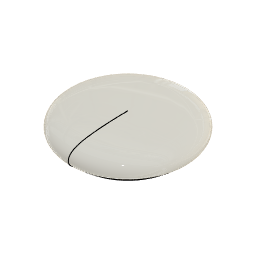
airtag (Autodesk Fusion 360 design; units mm, degrees)
Autodesk Fusion 360 part; units mm, degrees
sketch "airtag_guidelines" plane through (0, 0, 0) normal (1, 0, 0) x (0, 1, 0)
  spline S0 degree 5 poles (15.93, 7.98) (15.8968, 7.9797) (15.8305, 7.9792) (15.731, 7.9782) (15.5984, 7.9768) (15.4326, 7.9748) (15.2668, 7.9725) (15.1011, 7.97) (14.9353, 7.9675) (14.7696, 7.9651) (14.6038, 7.963) (14.438, 7.9613) (14.2722, 7.9599) (14.1063, 7.9589) (13.9405, 7.9579) (13.7747, 7.9563) (13.6089, 7.954) (13.4432, 7.9504) (13.2776, 7.9456) (13.112, 7.9397) (12.9463, 7.9332) (12.7805, 7.9265) (12.6146, 7.9201) (12.4485, 7.9141) (12.2825, 7.9085) (12.1166, 7.903) (11.951, 7.897) (11.7857, 7.8905) (11.6209, 7.883) (11.4563, 7.8749) (11.292, 7.8664) (11.1275, 7.858) (10.9629, 7.85) (10.7979, 7.8425) (10.6324, 7.8353) (10.4666, 7.8278) (10.3005, 7.8198) (10.1343, 7.8106) (9.9681, 7.8001) (9.802, 7.7884) (9.6363, 7.7759) (9.471, 7.7631) (9.3062, 7.7504) (9.1418, 7.7381) (8.9776, 7.7262) (8.8134, 7.7145) (8.6489, 7.7027) (8.484, 7.6905) (8.3185, 7.6776) (8.1528, 7.664) (7.9869, 7.6499) (7.8213, 7.6354) (7.6561, 7.6206) (7.4914, 7.6056) (7.3272, 7.5903) (7.1632, 7.5745) (6.9991, 7.5581) (6.8346, 7.5407) (6.6697, 7.5224) (6.5043, 7.5031) (6.3387, 7.483) (6.1733, 7.4623) (6.0081, 7.4411) (5.8435, 7.4197) (5.6793, 7.3981) (5.5155, 7.3762) (5.3518, 7.354) (5.1881, 7.3313) (5.0242, 7.3079) (4.8602, 7.2835) (4.6963, 7.2579) (4.5325, 7.2308) (4.369, 7.2021) (4.2061, 7.1716) (4.0436, 7.1393) (3.8817, 7.1053) (3.7201, 7.0696) (3.5589, 7.0325) (3.3981, 6.9939) (3.2375, 6.9538) (3.0773, 6.9121) (2.9176, 6.8686) (2.7585, 6.8231) (2.6001, 6.7754) (2.4426, 6.7249) (2.2861, 6.6715) (2.1309, 6.6147) (1.977, 6.5541) (1.8247, 6.4894) (1.6742, 6.4204) (1.5257, 6.3469) (1.3795, 6.2687) (1.2359, 6.1854) (1.0956, 6.0968) (0.9593, 6.0023) (0.8277, 5.9012) (0.7019, 5.793) (0.583, 5.6772) (0.472, 5.5536) (0.37, 5.4222) (0.2781, 5.2835) (0.1973, 5.138) (0.1288, 4.9864) (0.0733, 4.8296) (0.0316, 4.6687) (0.0046, 4.5046) (-0.0074, 4.3386) (-0.004, 4.172) (0.0148, 4.0061) (0.0489, 3.8424) (0.0977, 3.6825) (0.1605, 3.5277) (0.2364, 3.3793) (0.3243, 3.238) (0.4228, 3.1043) (0.5307, 2.9782) (0.6465, 2.8595) (0.7691, 2.7478) (0.8975, 2.643) (1.0309, 2.5447) (1.1691, 2.4529) (1.2832, 2.3846) (1.3708, 2.3362) (1.4301, 2.3052) (1.46, 2.29) knots 0 0 0 0 0 0 0.00833333 0.01666667 0.025 0.03333333 0.04166667 0.05 0.05833333 0.06666667 0.075 0.08333333 0.09166667 0.1 0.10833333 0.11666667 0.125 0.13333333 0.14166667 0.15 0.15833333 0.16666667 0.175 0.18333333 0.19166667 0.2 0.20833333 0.21666667 0.225 0.23333333 0.24166667 0.25 0.25833333 0.26666667 0.275 0.28333333 0.29166667 0.3 0.30833333 0.31666667 0.325 0.33333333 0.34166667 0.35 0.35833333 0.36666667 0.375 0.38333333 0.39166667 0.4 0.40833333 0.41666667 0.425 0.43333333 0.44166667 0.45 0.45833333 0.46666667 0.475 0.48333333 0.49166667 0.5 0.50833333 0.51666667 0.525 0.53333333 0.54166667 0.55 0.55833333 0.56666667 0.575 0.58333333 0.59166667 0.6 0.60833333 0.61666667 0.625 0.63333333 0.64166667 0.65 0.65833333 0.66666667 0.675 0.68333333 0.69166667 0.7 0.70833333 0.71666667 0.725 0.73333333 0.74166667 0.75 0.75833333 0.76666667 0.775 0.78333333 0.79166667 0.8 0.80833333 0.81666667 0.825 0.83333333 0.84166667 0.85 0.85833333 0.86666667 0.875 0.88333333 0.89166667 0.9 0.90833333 0.91666667 0.925 0.93333333 0.94166667 0.95 0.95833333 0.96666667 0.975 0.98333333 0.99166667 1 1 1 1 1 1
  spline S1 degree 5 poles (3.21, 0.88) (3.2486, 0.8746) (3.3257, 0.8637) (3.4417, 0.8476) (3.5967, 0.8264) (3.791, 0.8004) (3.9858, 0.7748) (4.1811, 0.7497) (4.3768, 0.7251) (4.5727, 0.7008) (4.7684, 0.6769) (4.9639, 0.6533) (5.1589, 0.6301) (5.3535, 0.6071) (5.5478, 0.5846) (5.742, 0.5624) (5.9363, 0.5408) (6.131, 0.5198) (6.3261, 0.4992) (6.5217, 0.4791) (6.7176, 0.4592) (6.9136, 0.4395) (7.1096, 0.42) (7.3055, 0.4006) (7.5011, 0.3817) (7.6968, 0.3634) (7.8925, 0.346) (8.0885, 0.3298) (8.2846, 0.3148) (8.4808, 0.3007) (8.6769, 0.2872) (8.8728, 0.2738) (9.0682, 0.2602) (9.2632, 0.2462) (9.4579, 0.2319) (9.6524, 0.2175) (9.847, 0.2033) (10.0419, 0.1897) (10.2372, 0.1768) (10.4329, 0.1645) (10.6291, 0.1527) (10.8255, 0.1412) (11.0219, 0.1299) (11.2183, 0.1186) (11.4145, 0.1076) (11.6105, 0.0972) (11.8063, 0.0878) (12.002, 0.0796) (12.1977, 0.0726) (12.3934, 0.0666) (12.5894, 0.0612) (12.7857, 0.0558) (12.9824, 0.05) (13.1795, 0.0438) (13.3769, 0.0372) (13.5743, 0.0307) (13.7717, 0.0247) (13.9688, 0.0197) (14.1655, 0.0159) (14.3618, 0.0134) (14.5578, 0.0118) (14.7536, 0.0108) (14.9493, 0.01) (15.1451, 0.0091) (15.341, 0.0078) (15.5371, 0.0059) (15.6942, 0.0038) (15.812, 0.002) (15.8907, 0.0007) (15.93, 0) knots 0 0 0 0 0 0 0.01538462 0.03076923 0.04615385 0.06153846 0.07692308 0.09230769 0.10769231 0.12307692 0.13846154 0.15384615 0.16923077 0.18461538 0.2 0.21538462 0.23076923 0.24615385 0.26153846 0.27692308 0.29230769 0.30769231 0.32307692 0.33846154 0.35384615 0.36923077 0.38461538 0.4 0.41538462 0.43076923 0.44615385 0.46153846 0.47692308 0.49230769 0.50769231 0.52307692 0.53846154 0.55384615 0.56923077 0.58461538 0.6 0.61538462 0.63076923 0.64615385 0.66153846 0.67692308 0.69230769 0.70769231 0.72307692 0.73846154 0.75384615 0.76923077 0.78461538 0.8 0.81538462 0.83076923 0.84615385 0.86153846 0.87692308 0.89230769 0.90769231 0.92307692 0.93846154 0.95384615 0.96923077 0.98461538 1 1 1 1 1 1
  line L0 (3.205, 1.89) -> (15.93, 1.89)
  line L1 (15.93, 1.89) -> (15.93, 0.88)
  line L2 (15.93, 0.88) -> (3.205, 0.88)
  line L3 (3.155, 0.93) -> (3.155, 1.84)
  line L4 (15.93, 7.98) -> (15.93, 0)
  line L5 (4.375, 2.29) -> (15.93, 2.29)
  line L6 (15.93, 2.29) -> (15.93, 1.89)
  line L7 (15.93, 1.89) -> (4.375, 1.89)
  line L8 (4.375, 1.89) -> (4.375, 2.29)
  line L9 (1.46, 2.29) -> (4.375, 2.29)
  line L10 (3.205, 1.89) -> (3.155, 1.84)
  line L11 (3.205, 0.88) -> (3.155, 0.93)
  point P0 (15.93, 0)
  point P1 (14.95, 0.01)
  point P2 (13.97, 0.02)
  point P3 (12.98, 0.05)
  point P4 (12, 0.08)
  point P5 (11.02, 0.13)
  point P6 (10.04, 0.19)
  point P7 (9.07, 0.26)
  point P8 (0.77, 2.75)
  point P9 (1.46, 2.29)
  point P10 (3.21, 0.88)
  point P11 (4.18, 0.75)
  point P12 (5.16, 0.63)
  point P13 (6.13, 0.52)
  point P14 (7.11, 0.42)
  point P15 (8.09, 0.33)
  point P16 (13.44, 7.95)
  point P17 (14.27, 7.96)
  point P18 (0.58, 5.67)
  point P19 (0.13, 4.98)
  point P20 (0.24, 3.38)
  point P21 (0, 4.17)
  point P22 (15.93, 7.98)
  point P23 (15.1, 7.97)
  point P24 (6.83, 7.54)
  point P25 (7.65, 7.62)
  point P26 (8.48, 7.69)
  point P27 (9.3, 7.75)
  point P28 (10.13, 7.81)
  point P29 (10.96, 7.85)
  point P30 (11.78, 7.89)
  point P31 (12.61, 7.92)
  point P32 (1.97, 6.55)
  point P33 (2.75, 6.82)
  point P34 (3.55, 7.03)
  point P35 (4.36, 7.2)
  point P36 (5.18, 7.33)
  point P37 (6, 7.44)
  point P38 (1.23, 6.18)
  point P39 (15.1, 7.97)
  point P40 (14.27, 7.96)
  point P41 (13.44, 7.95)
  point P42 (12.61, 7.92)
  point P43 (11.78, 7.89)
  point P44 (10.96, 7.85)
  point P45 (10.13, 7.81)
  point P46 (9.3, 7.75)
  point P47 (8.48, 7.69)
  point P48 (7.65, 7.62)
  point P49 (6.83, 7.54)
  point P50 (6, 7.44)
  point P51 (5.18, 7.33)
  point P52 (4.36, 7.2)
  point P53 (3.55, 7.03)
  point P54 (2.75, 6.82)
  point P55 (1.97, 6.55)
  point P56 (1.23, 6.18)
  point P57 (0.58, 5.67)
  point P58 (0.13, 4.98)
  point P59 (0, 4.17)
  point P60 (0.24, 3.38)
  point P61 (0.77, 2.75)
  point P62 (4.18, 0.75)
  point P63 (5.16, 0.63)
  point P64 (6.13, 0.52)
  point P65 (7.11, 0.42)
  point P66 (8.09, 0.33)
  point P67 (9.07, 0.26)
  point P68 (10.04, 0.19)
  point P69 (11.02, 0.13)
  point P70 (12, 0.08)
  point P71 (12.98, 0.05)
  point P72 (13.97, 0.02)
  point P73 (14.95, 0.01)
  point P74 (3.155, 1.89)
  point P75 (3.155, 0.88)
  dimension "d4_1" = 15.93
  dimension "d5_1" = 14.95
  dimension "d6_1" = 0.01
  dimension "d7_1" = 13.97
  dimension "d8_1" = 0.02
  dimension "d9_1" = 12.98
  dimension "d10_1" = 0.05
  dimension "d11_1" = 12
  dimension "d12_1" = 0.08
  dimension "d13_1" = 11.02
  dimension "d14_1" = 0.13
  dimension "d15_1" = 10.04
  dimension "d16_1" = 0.19
  dimension "d17_1" = 9.07
  dimension "d18_1" = 0.26
  dimension "d19_1" = 8.09
  dimension "d20_1" = 0.33
  dimension "d21_1" = 7.11
  dimension "d22_1" = 0.42
  dimension "d23_1" = 6.13
  dimension "d24_1" = 0.52
  dimension "d25_1" = 5.16
  dimension "d26_1" = 0.63
  dimension "d27_1" = 4.18
  dimension "d28_1" = 0.75
  dimension "d29_1" = 3.21
  dimension "d30_1" = 0.88
  dimension "d31_1" = 1.46
  dimension "d32_1" = 2.29
  dimension "d33_1" = 0.77
  dimension "d34_1" = 2.75
  dimension "d35_1" = 0.24
  dimension "d36_1" = 3.38
  dimension "d37_1" = 4.17
  dimension "d38_1" = 0.13
  dimension "d39_1" = 4.98
  dimension "d40_1" = 0.58
  dimension "d41_1" = 5.67
  dimension "d42_1" = 15.93
  dimension "d43_1" = 7.98
  dimension "d44_1" = 15.1
  dimension "d45_1" = 7.97
  dimension "d46_1" = 14.27
  dimension "d47_1" = 7.96
  dimension "d48_1" = 13.44
  dimension "d49_1" = 7.95
  dimension "d50_1" = 12.61
  dimension "d51_1" = 7.92
  dimension "d52_1" = 11.78
  dimension "d53_1" = 7.89
  dimension "d54_1" = 10.96
  dimension "d55_1" = 7.85
  dimension "d56_1" = 10.13
  dimension "d57_1" = 7.81
  dimension "d58_1" = 9.3
  dimension "d59_1" = 7.75
  dimension "d60_1" = 8.48
  dimension "d61_1" = 7.69
  dimension "d62_1" = 7.65
  dimension "d63_1" = 7.62
  dimension "d64_1" = 6.83
  dimension "d65_1" = 7.54
  dimension "d66_1" = 6
  dimension "d67_1" = 7.44
  dimension "d68_1" = 5.18
  dimension "d69_1" = 7.33
  dimension "d70_1" = 4.36
  dimension "d71_1" = 7.2
  dimension "d72_1" = 3.55
  dimension "d73_1" = 7.03
  dimension "d74_1" = 2.75
  dimension "d75_1" = 6.82
  dimension "d76_1" = 1.97
  dimension "d77_1" = 6.55
  dimension "d78_1" = 1.23
  dimension "d79_1" = 6.18
  dimension "d80_1" = 12.775
  dimension "d81_1" = 1.01
  dimension "d82_1" = 11.555
  dimension "d83_1" = 0.4
  dimension "d84_1" = 0.05
  dimension "d85_1" = 0.05
  dimension "d86_1" = 0.05
  dimension "d87_1" = 0.05
  constraint horizontal origin S1.end
  constraint vertical origin P59
  constraint coincident P22 S0.start
  constraint coincident P39 P23
  constraint coincident P40 P17
  constraint coincident P41 P16
  constraint coincident P42 P31
  constraint coincident P43 P30
  constraint coincident P44 P29
  constraint coincident P45 P28
  constraint coincident P46 P27
  constraint coincident P47 P26
  constraint coincident P48 P25
  constraint coincident P49 P24
  constraint coincident P50 P37
  constraint coincident P51 P36
  constraint coincident P52 P35
  constraint coincident P53 P34
  constraint coincident P54 P33
  constraint coincident P55 P32
  constraint coincident P56 P38
  constraint coincident P57 P18
  constraint coincident P58 P19
  constraint coincident P59 P21
  constraint coincident P60 P20
  constraint coincident P61 P8
  constraint coincident P9 S0.end
  constraint coincident P10 S1.start
  constraint coincident P62 P11
  constraint coincident P63 P12
  constraint coincident P64 P13
  constraint coincident P65 P14
  constraint coincident P66 P15
  constraint coincident P67 P7
  constraint coincident P68 P6
  constraint coincident P69 P5
  constraint coincident P70 P4
  constraint coincident P71 P3
  constraint coincident P72 P2
  constraint coincident P73 P1
  constraint coincident P0 S1.end
  constraint horizontal L0
  constraint vertical L1
  constraint horizontal L2
  constraint vertical L3
  constraint collinear L1 L4
  constraint coincident P10 L2
  constraint horizontal L5
  constraint vertical L6
  constraint horizontal L7
  constraint vertical L8
  constraint collinear L4 L6
  constraint collinear L0 L7
  constraint coincident P74 L0
  constraint coincident P74 L3
  constraint coincident P75 L2
  constraint coincident P75 L3
  measures "d4_1" distance of origin S1.end
  measures "d5_1" horizontal distance of origin P73
  measures "d6_1" vertical distance of origin P73
  measures "d7_1" horizontal distance of origin P72
  measures "d8_1" vertical distance of origin P72
  measures "d9_1" horizontal distance of origin P71
  measures "d10_1" vertical distance of origin P71
  measures "d11_1" horizontal distance of origin P70
  measures "d12_1" vertical distance of origin P70
  measures "d13_1" horizontal distance of origin P69
  measures "d14_1" vertical distance of origin P69
  measures "d15_1" horizontal distance of origin P68
  measures "d16_1" vertical distance of origin P68
  measures "d17_1" horizontal distance of origin P67
  measures "d18_1" vertical distance of origin P67
  measures "d19_1" horizontal distance of origin P66
  measures "d20_1" vertical distance of origin P66
  measures "d21_1" horizontal distance of origin P65
  measures "d22_1" vertical distance of origin P65
  measures "d23_1" horizontal distance of origin P64
  measures "d24_1" vertical distance of origin P64
  measures "d25_1" horizontal distance of origin P63
  measures "d26_1" vertical distance of origin P63
  measures "d27_1" horizontal distance of origin P62
  measures "d28_1" vertical distance of origin P62
  measures "d29_1" horizontal distance of origin P10
  measures "d30_1" vertical distance of origin P10
  measures "d31_1" horizontal distance of origin P9
  measures "d32_1" vertical distance of origin P9
  measures "d33_1" horizontal distance of origin P61
  measures "d34_1" vertical distance of origin P61
  measures "d35_1" horizontal distance of origin P60
  measures "d36_1" vertical distance of origin P60
  measures "d37_1" vertical distance of origin P59
  measures "d38_1" horizontal distance of origin P58
  measures "d39_1" vertical distance of origin P58
  measures "d40_1" horizontal distance of origin P57
  measures "d41_1" vertical distance of origin P57
  measures "d42_1" horizontal distance of origin P22
  measures "d43_1" vertical distance of origin P22
  measures "d44_1" horizontal distance of origin P39
  measures "d45_1" vertical distance of origin P39
  measures "d46_1" horizontal distance of origin P40
  measures "d47_1" vertical distance of origin P40
  measures "d48_1" horizontal distance of origin P41
  measures "d49_1" vertical distance of origin P41
  measures "d50_1" horizontal distance of origin P42
  measures "d51_1" vertical distance of origin P42
  measures "d52_1" horizontal distance of origin P43
  measures "d53_1" vertical distance of origin P43
  measures "d54_1" horizontal distance of origin P44
  measures "d55_1" vertical distance of origin P44
  measures "d56_1" horizontal distance of origin P45
  measures "d57_1" vertical distance of origin P45
  measures "d58_1" horizontal distance of origin P46
  measures "d59_1" vertical distance of origin P46
  measures "d60_1" horizontal distance of origin P47
  measures "d61_1" vertical distance of origin P47
  measures "d62_1" horizontal distance of origin P48
  measures "d63_1" vertical distance of origin P48
  measures "d64_1" horizontal distance of origin P49
  measures "d65_1" vertical distance of origin P49
  measures "d66_1" horizontal distance of origin P50
  measures "d67_1" vertical distance of origin P50
  measures "d68_1" horizontal distance of origin P51
  measures "d69_1" vertical distance of origin P51
  measures "d70_1" horizontal distance of origin P52
  measures "d71_1" vertical distance of origin P52
  measures "d72_1" horizontal distance of origin P53
  measures "d73_1" vertical distance of origin P53
  measures "d74_1" horizontal distance of origin P54
  measures "d75_1" vertical distance of origin P54
  measures "d76_1" horizontal distance of origin P55
  measures "d77_1" vertical distance of origin P55
  measures "d78_1" horizontal distance of origin P56
  measures "d79_1" vertical distance of origin P56
  measures "d80_1" distance of P74 L0.end
  measures "d81_1" distance of P74 P75
  measures "d82_1" distance of L5.start L5.end
  measures "d83_1" distance of L5.start L7.end
  measures "d84_1" distance of P74 L0.start
  measures "d85_1" distance of P74 L3.end
  measures "d86_1" distance of P75 L2.end
  measures "d87_1" distance of P75 L3.start
revolve "Revolve1" add sketch "airtag_guidelines" angle 360 about axis through (0, 15.93, 7.98) along (0, 0, -1) contours S0 L4 L5 L9 makes body 1
revolve "Revolve2" add sketch "airtag_guidelines" angle 360 about axis through (0, 15.93, 7.98) along (0, 0, -1) separate body contours L0 L4 L5 L6 L7 L8 | L0 L1 L2 L3 L4 L7 L10 L11 | S1 L2 L4 makes body 2
equation "d80_1 = ( 25.55 / 2 ) * 1 mm"
equation "d81_1 = 1.89 mm - 0.88 mm"
equation "d82_1 = ( 23.11 / 2 ) * 1 mm"
equation "d83_1 = 2.29 mm - 1.89 mm"
equation "d85_1 = d84_1"
equation "d87_1 = d86_1"
named bodies: "plastic", "metal"
